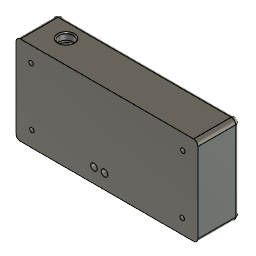
heltec-wp-gehaeuse (Autodesk Fusion 360 design; units mm, degrees)
Autodesk Fusion 360 part; units mm, degrees
sketch "Skizze1" plane through (0, 0, 0) normal (0, 1, 0) x (1, 0, 0)
  line L0 (0, 0) -> (72.1, 0)
  line L1 (72.1, 0) -> (72.1, -30)
  line L2 (72.1, -30) -> (0, -30)
  line L3 (0, -30) -> (0, 0)
  dimension "d1" = 72.1
  dimension "d2" = 30
  constraint horizontal L0
  constraint vertical L1
  constraint horizontal L2
  constraint vertical L3
  constraint coincident L0.start L3.end
  measures "d1" distance of L0.start L0.end
  measures "d2" distance of L0.start L2.end
extrude "Extrusion3" add sketch "Skizze1" along normal blind 14
shell "Schale3" thickness 5 outward yes removed faces 1 at (24.0333, 14, 20)
fillet "Abrundung1" radius 2 1 edges at (77.1, 4.5, 35)
fillet "Abrundung2" radius 2 8 edges at (36.05, 14, -5) (-5, 14, 15) (35.05, 14, 35) (76.5142, 14, 34.4142) (77.1, 14, 14) (-5, 4.5, 35) (-5, 4.5, -5) (77.1, 4.5, -5)
sketch "Skizze3" plane through (-5, 0, 0) normal (-1, 0, 0) x (0, -1, 0)
  line L0 (5, 33) -> (-12, 33)
  line L1 (-12, 33) -> (-12, -3)
  line L2 (-12, -3) -> (5, -3)
  line L3 (5, -3) -> (5, 33)
  line L4 (-6.5193, 0.3431, -0.3618) -> (-4.5193, 0.3431, -0.3618)
  line L5 (-1.5193, 3.3431, -0.3618) -> (-1.5193, 13.3431, -0.3618)
  line L6 (-4.5193, 16.3431, -0.3618) -> (-6.5193, 16.3431, -0.3618)
  line L7 (-9.5193, 13.3431, -0.3618) -> (-9.5193, 3.3431, -0.3618)
  arc A0 through (-6.5193, 16.3431, -0.3618) (-8.6406, 15.4644, -0.3618) (-9.5193, 13.3431, -0.3618)
  arc A1 through (-1.5193, 13.3431, -0.3618) (-2.398, 15.4644, -0.3618) (-4.5193, 16.3431, -0.3618)
  arc A2 through (-4.5193, 0.3431, -0.3618) (-2.398, 1.2217, -0.3618) (-1.5193, 3.3431, -0.3618)
  arc A3 through (-9.5193, 3.3431, -0.3618) (-8.6406, 1.2217, -0.3618) (-6.5193, 0.3431, -0.3618)
  point P0 (-9.5193, 0.3431)
  point P1 (-1.5193, 0.3431)
  point P2 (-9.5193, 16.3431)
  dimension "d19" = 8
  dimension "d20" = 16
  dimension "d67" = 3
  measures "d19" distance of P0 P1
  measures "d20" distance of P0 P2
extrude "Extrusion4" cut sketch "Skizze3" along normal blind 30 contours L4 L5 L6 L7 A0 A1 A2 A3 in plane through (-4.6382, 0, 0) normal (-1, 0, 0)
sketch "Skizze4" plane through (0, 0, 0) normal (0, 1, 0) x (1, 0, 0)
  line L0 (67.4387, -27.7344) -> (4.3603, -27.7344)
  line L1 (4.3603, -27.7344) -> (4.3603, -3.1975)
  line L2 (4.3603, -3.1975) -> (67.4387, -3.1975)
  line L3 (67.4387, -3.1975) -> (67.4387, -27.7344)
  constraint horizontal L0
  constraint vertical L1
  constraint horizontal L2
  constraint vertical L3
extrude "Extrusion5" cut sketch "Skizze4" against normal blind 3.5
sketch "Skizze5" plane through (0, 0, 0) normal (0, 1, 0) x (1, 0, 0)
hole "Bohrung2" at (2.2015, 0, 2.0351) direction (0, -1, 0) diameter 2 depth 9 tip angle 118
hole "Bohrung3" at (69.984, 0, 1.6) direction (0, -1, 0) diameter 2 depth 9 tip angle 118
hole "Bohrung4" at (1.8713, 0, 27.9375) direction (0, -1, 0) diameter 2 depth 9 tip angle 118
hole "Bohrung5" at (70.2795, 0, 27.9919) direction (0, -1, 0) diameter 2 depth 9 tip angle 118
extrude "Extrusion6" cut 1 faces at (-4.6382, 4.1859, 10.0097) along direction (1, 0, 0) blind 20
hole "Bohrung6" at (7.1183, 5.5048, 35) direction (0, 0, -1) diameter 6.5 depth 15 tip angle 118
sketch "Skizze6" plane through (0, 0, 30) normal (0, 0, -1) x (1, 0, 0)
  circle A0 centre (7.1183, -5.5048) radius 3.25
  line L0 (72.1, 0) -> (0, 0)
  line L1 (0, 0) -> (0, -14)
  line L2 (0, -14) -> (72.1, -14)
  line L3 (72.1, -14) -> (72.1, 0)
  circle A1 centre (7.1183, -5.5048) radius 4.7717
  constraint concentric A0 A1
extrude "Extrusion7" cut sketch "Skizze6" against normal blind 2 contours A1
fillet "Abrundung3" radius 0.5 1 edges at (4.0882, 6.68, 35)
fillet "Abrundung4" radius 0.5 4 edges at (-5, 5.5193, 16.3431) (-5, 1.5193, 8.3431) (0, 5.5193, 0.3431) (-5, 9.5193, 8.3431)
sketch "Skizze7" plane through (77.1, 0, 0) normal (1, 0, 0) x (0, 1, 0)
  line L0 (12, -3) -> (12, 33)
  line L1 (12, 33) -> (-5, 33)
  line L2 (-5, 33) -> (-5, -3)
  line L3 (-5, -3) -> (12, -3)
sketch "Skizze8" plane through (0, 0, 0) normal (0, 1, 0) x (1, 0, 0)
  line L0 (45, -3) -> (14.5333, -3)
  line L1 (14.5333, -3) -> (14.5333, 0.0407)
  line L2 (14.5333, 0.0407) -> (45, 0.0407)
  line L3 (45, 0.0407) -> (45, -3)
  constraint horizontal L0
  constraint vertical L1
  constraint horizontal L2
  constraint vertical L3
extrude "Extrusion8" cut sketch "Skizze8" along normal blind 4
sketch "Skizze9" plane through (0, 0, 0) normal (0, 1, 0) x (1, 0, 0)
  line L0 (46.4497, -3.1754) -> (14, -3.1754)
  line L1 (14, -3.1754) -> (14, 0)
  line L2 (14, 0) -> (46.4497, 0)
  line L3 (46.4497, 0) -> (46.4497, -3.1754)
  constraint horizontal L0
  constraint vertical L1
  constraint horizontal L2
  constraint vertical L3
extrude "Extrusion9" add sketch "Skizze9" along normal blind 3
hole "Bohrung7" at (30.2249, 3, 1.5877) direction (0, -1, 0) diameter 3 depth 10 tip angle 118
hole "Bohrung8" at (34.9432, 3, 1.6156) direction (0, -1, 0) diameter 3 depth 10 tip angle 118
sketch "Skizze11" plane through (0, 3, 0) normal (0, 1, 0) x (-1, 0, 0)
  circle A0 centre (-34.9432, 1.6156) radius 1.5
  circle A1 centre (-30.2249, 1.5877) radius 1.5
  line L0 (-46.4497, 0) -> (-45, 0)
  line L1 (-45, 0) -> (-14.5333, 0)
  line L2 (-14.5333, 0) -> (-14, 0)
  line L3 (-14, 0) -> (-14, 3.1754)
  line L4 (-14, 3.1754) -> (-46.4497, 3.1754)
  line L5 (-46.4497, 3.1754) -> (-46.4497, 0)
  line L6 (-38.6742, 3.1754) -> (-26.6742, 3.1754)
  line L7 (-26.6742, 3.1754) -> (-26.6742, 0.1754)
  line L8 (-26.6742, 0.1754) -> (-38.6742, 0.1754)
  line L9 (-38.6742, 0.1754) -> (-38.6742, 3.1754)
  dimension "d59" = 12
  dimension "d60" = 3
  constraint horizontal L6
  constraint vertical L7
  constraint horizontal L8
  constraint vertical L9
  constraint coincident L4 L6.start
  measures "d59" distance of L6.start L6.end
  measures "d60" distance of L6.start L8.end
extrude "Extrusion10" cut sketch "Skizze11" against normal blind 2 contours A0 A1 L4 L6 L7 L8 L9
extrude "Extrusion11" add 1 faces at (53.446, 0, 2.1243) along direction (0, 1, 0) blind 2
extrude "Extrusion12" cut 1 faces at (2.9068, 2, 15.5682) along direction (0, -1, 0) blind 1
